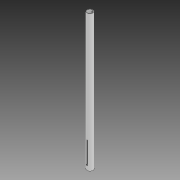
# Autodesk Inventor part: FE-120-007 Door Tube
Saved by Autodesk Inventor 2021 (Build 250183000, 183)
## iProperties
Created: 2021-01-11
Part Number: FE-120-007 Door Tube
Material: Aluminum 6061
Document SubType Name: Modeling
Density: 2.7 g/cm^3
Appearance: Aluminum - Dark
Autodesk Inventor part; units mm, degrees
ref_plane "YZ Plane" through (0, 0, 0) normal (1, 0, 0) x (0, 1, 0)
ref_plane "XZ Plane" through (0, 0, 0) normal (0, 1, 0) x (-1, 0, 0)
ref_plane "XY Plane" through (0, 0, 0) normal (0, 0, 1) x (1, 0, 0)
sketch "Sketch1" plane through (0, 0, 0) normal (0, 1, 0) x (-1, 0, 0)
  circle A0 centre (0, 0) radius 21.082
  circle A1 centre (0, 0) radius 17.526
  dimension "d0" = 42.164
  dimension "d1" = 35.052
  constraints: 2 centre point, 2 coincident
  measures "d0" diameter of A0
  measures "d1" diameter of A1
extrude "Extrusion1" add sketch "Sketch1" along normal mid plane 965.2
sketch "Sketch3" plane through (0, 0, 0) normal (0, 0, 1) x (1, 0, 0)
  line L0 (0, 474.6625) -> (0, 461.9625) construction
  line L1 (-3.175, 474.6625) -> (-3.175, 461.9625)
  line L2 (3.175, 461.9625) -> (3.175, 474.6625)
  arc A0 (3.175, 474.6625) -> (-3.175, 474.6625) centre (0, 474.6625) ccw
  arc A1 (-3.175, 461.9625) -> (3.175, 461.9625) centre (0, 461.9625) ccw
  line L3 (0, 436.5625) -> (0, 423.8625) construction
  line L4 (-3.175, 436.5625) -> (-3.175, 423.8625)
  line L5 (3.175, 423.8625) -> (3.175, 436.5625)
  arc A2 (3.175, 436.5625) -> (-3.175, 436.5625) centre (0, 436.5625) ccw
  arc A3 (-3.175, 423.8625) -> (3.175, 423.8625) centre (0, 423.8625) ccw
  line L6 (0, -298.45) -> (0, -450.85) construction
  line L7 (-3.175, -298.45) -> (-3.175, -450.85)
  line L8 (3.175, -450.85) -> (3.175, -298.45)
  arc A4 (3.175, -298.45) -> (-3.175, -298.45) centre (0, -298.45) ccw
  arc A5 (-3.175, -450.85) -> (3.175, -450.85) centre (0, -450.85) ccw
  line L9 (0, -450.85) -> (-6.35, -450.85) construction
  line L10 (0, -447.675) -> (-6.35, -447.675)
  line L11 (-6.35, -454.025) -> (0, -454.025)
  arc A6 (0, -454.025) -> (0, -447.675) centre (0, -450.85) ccw
  arc A7 (-6.35, -447.675) -> (-6.35, -454.025) centre (-6.35, -450.85) ccw
  line L12 (-21.082, -482.6) -> (21.082, -482.6) projected
  line L13 (21.082, 482.6) -> (-21.082, 482.6) projected
  point P0 (0, 468.3125)
  point P1 (0, 430.2125)
  point P2 (0, -374.65)
  point P3 (-3.175, -450.85)
  point P4 (0, -482.6)
  point P5 (-3.175, -447.675)
  dimension "d17" = 3.175
  dimension "d18" = 12.7
  dimension "d19" = 6.35
  dimension "d20" = 152.4
  dimension "d21" = 28.575
  dimension "d22" = 25.4
  dimension "d23" = 7.9375
  constraints: 32 end point, 16 point on circle, 16 tangent, 8 centre point, 5 midpoint, 4 parallel, 3 equal radius, 2 collinear, 2 point on line, 2 vertical, 1 perpendicular, 1 vertical alignment
  measures "d17" radius of A0
  measures "d18" distance of L0.start L0.end
  measures "d19" distance of L6.end L9.end
  measures "d20" distance of L6.start L6.end
  measures "d21" distance between parallel lines of L12 L11
  measures "d22" distance of L0.end L3.start
  measures "d23" distance from line of L0.start L13
extrude "Extrusion3" cut sketch "Sketch3" against normal through all contours A0 L2 A1 L1 | A2 L5 A3 L4
extrude "Extrusion4" cut sketch "Sketch3" along normal blind 25.4 contours A4 L8 A6 L10 L7 | L10 A6 A5 L7 | L7 A5 L11 A7 L10
body "Solid1"
